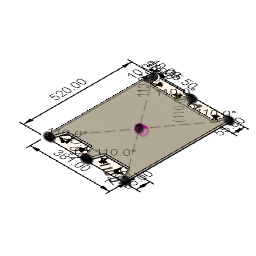
1-Cold Build Plate v3 (Autodesk Fusion 360 design; units mm, degrees)
Autodesk Fusion 360 part; units mm, degrees
note: some values were not read from the file. Chosen so that the rebuilt part matches the saved one: that a step has no effect; which face or edge a step refers to. Set by a fixed rule: which sketch regions a step uses.
mesh "Mesh1" [no effect]
sketch "Mesh Section Sketch XY" plane through (0, 0, 5) normal (0, 0, 1) x (1, 0, 0)
mesh "Mesh2" [no effect]
sketch "Mesh Section Sketch XY V3" plane through (0, 0, 20) normal (0, 0, 1) x (1, 0, 0)
sketch "Mesh Section Sketch XZ V3" plane through (0, 0, 0) normal (0, 1, 0) x (-1, 0, 0)
sketch "Sketch2" plane through (0, 0, 0) normal (0, 0, 1) x (1, 0, 0)
  line L0 (190.5, -260) -> (-190.5, -260)
  line L1 (-190.5, -260) -> (-190.5, 260)
  line L2 (-190.5, 260) -> (190.5, 260)
  line L3 (190.5, 260) -> (190.5, -260)
  line L4 (190.5, -260) -> (-190.5, 260) construction
  line L5 (-190.5, -260) -> (190.5, 260) construction
  line L6 (-153.4796, 205) -> (153.4796, 205)
  line L7 (149.8399, -195) -> (-149.8399, -195)
  circle A0 centre (-180.5, 250) radius 2.75
  line L8 (-171.823, 255.3981) -> (-153.4796, 205)
  circle A1 centre (0, 250) radius 2.75
  circle A2 centre (180.5, 250) radius 2.75
  circle A3 centre (-180.5, -250) radius 2.75
  circle A4 centre (0, -250) radius 2.75
  circle A5 centre (180.5, -250) radius 2.75
  arc A6 (-170.5, 250) -> (-190.5, 250) centre (-180.5, 250) ccw
  line L9 (-180.5, 250) -> (-170.5, 250) construction
  line L10 (-180.5, 250) -> (-190.5, 250) construction
  arc A7 (10, 250) -> (-10, 250) centre (0, 250) ccw
  arc A8 (190.5, 250) -> (170.5, 250) centre (180.5, 250) ccw
  line L11 (-27.0204, 205) -> (-9.3969, 253.4202)
  line L12 (9.3969, 253.4202) -> (27.0204, 205)
  line L13 (20, 0) -> (2.5, 0)
  arc A9 (-190.5, -250) -> (-170.5, -250) centre (-180.5, -250) ccw
  line L14 (-30.6601, -195) -> (-9.3969, -253.4202)
  line L15 (9.3969, -253.4202) -> (30.6601, -195)
  arc A10 (-10, -250) -> (10, -250) centre (0, -250) ccw
  arc A11 (171.7415, -245.1742) -> (190.5, -250) centre (180.5, -250) ccw
  line L16 (173.8856, -257.5) -> (187.1144, -257.5)
  line L17 (173.8856, 257.5) -> (187.1144, 257.5)
  line L18 (-149.8399, -195) -> (-171.1031, -253.4202)
  line L19 (153.4796, 205) -> (171.1031, 253.4202)
  line L20 (149.8399, -195) -> (171.1031, -253.4202)
  dimension "d1" = 381
  dimension "d2" = 520
  dimension "d5" = 5.5
  dimension "d6" = 10
  dimension "d7" = 10
  dimension "d10" = 361
  dimension "d11" = -500
  dimension "d12" = 180
  dimension "d14" = 110
  dimension "d17" = 7.5
  dimension "d18" = 65
  dimension "d19" = 55
  dimension "d23" = 110
  dimension "d24" = 110
  dimension "d30" = 110
  dimension "d31" = 110
  dimension "d32" = 110
  dimension "d35" = 110
  dimension "d36" = 110
  constraint perpendicular L0 L1
  constraint parallel L0 L2
  constraint parallel L1 L3
  constraint horizontal L0
  constraint coincident L4 origin
  constraint coincident L5 origin
  constraint parallel L6 L7
  constraint horizontal L6
  constraint coincident L1 A6.end
  constraint coincident A0.centre A6.centre
  constraint tangent L8 A6
  constraint coincident L6 L11.start
  constraint coincident A7 L11.end
  constraint coincident A7 L12.start
  constraint coincident L6 L12.end
  constraint tangent A7 L12
  constraint tangent A7 L11
  constraint equal L11 L12
  constraint horizontal L9
  constraint symmetric A6.start L13 A9.end
  constraint symmetric A6.end L13 A9.start
  constraint symmetric A6 L13 A9
  constraint symmetric A7.start L13 A10.end
  constraint symmetric A7.end L13 A10.start
  constraint symmetric A7 L13 A10
  constraint symmetric A8.start L13 A11.end
  constraint symmetric A8 L13 A11
  constraint symmetric L11.end L13 L14.end
  constraint symmetric L12.start L13 L15.start
  constraint coincident A11 L16.start
  constraint coincident A11 L16.end
  constraint parallel L0 L16
  constraint coincident A8 L17.start
  constraint coincident A8 L17.end
  constraint horizontal L17
  constraint symmetric L13 L16 L17
  constraint coincident L7 L14.start
  constraint coincident L7 L15.end
  constraint coincident A9 L18.end
  constraint tangent A9 L18
  constraint coincident A8 L19.end
  constraint tangent A8 L19
  constraint coincident A11 L20.end
  constraint tangent A11 L20
  measures "d1" distance of L0.start L0.end
  measures "d2" distance of L0.end L1.end
  measures "d5" diameter of A0
  measures "d6" distance of L1 A0.centre A1.centre
  measures "d7" distance of L2 A0.centre A1.centre
  measures "d12" angle of L9 L10
  measures "d14" angle of L6 L11
  measures "d17" distance of A5.centre L16
  measures "d18" distance of L0 L7
  measures "d19" distance of L2 L6
  measures "d23" angle of L7 L14
  measures "d24" angle of L7 L15
  measures "d30" angle of L6 L12
  measures "d31" angle of L6 L19
  measures "d32" angle of L7 L18
  measures "d35" angle of L6 L8
  measures "d36" angle of L7 L20
extrude "Extrude1" add sketch "Sketch2" along normal blind 10 contours L1 L3 L6 L7 L8 A6 A8 A9 A11 L16 L17 L18 L19 L20 | L7 L14 L15 A10 | L6 A7 L11 L12 | A2 | A5
fillet "Fillet1" radius 1.5 1 edges at (-190.5, 0, 10)
equation "d24 = d23"
